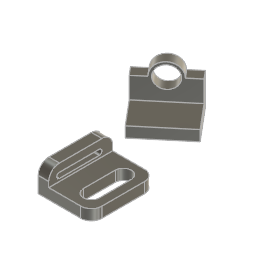
day-5 (Autodesk Fusion 360 design; units mm, degrees)
part number: 2026-04-15-21-22-57-199
Autodesk Fusion 360 part; units mm, degrees
sketch "Sketch1" plane through (0, 0, 0) normal (0, 0, 1) x (1, 0, 0)
  line L0 (0, 0) -> (100, 0)
  line L1 (100, 0) -> (100, -120)
  line L2 (100, -120) -> (0, -120)
  line L3 (0, -120) -> (0, 0)
  dimension "d1" = 100
  dimension "d2" = 120
  constraint horizontal L0
  constraint vertical L1
  constraint horizontal L2
  constraint vertical L3
  constraint coincident L0.start L3.end
  measures "d1" distance of L0.start L0.end
  measures "d2" distance of L0.start L2.end
extrude "Extrude1" add sketch "Sketch1" along normal blind 20 makes body 1
sketch "Sketch2" plane through (0, 0, 0) normal (0, 0, 1) x (1, 0, 0)
  line L0 (83.9736, -28.966) -> (83.9736, -88.966)
  line L1 (53.9736, -88.966) -> (53.9736, -28.966)
  arc A0 (83.9736, -28.966) -> (53.9736, -28.966) centre (68.9736, -28.966) ccw
  arc A1 (53.9736, -88.966) -> (83.9736, -88.966) centre (68.9736, -88.966) ccw
  constraint vertical L0
  constraint vertical L1
extrude "Extrude2" cut sketch "Sketch2" along normal blind 70 bodies 1
sketch "Sketch3" plane through (0, 0, 0) normal (0, 0, 1) x (1, 0, 0)
  line L0 (0, 0) -> (20, 0)
  line L1 (20, 0) -> (20, -120)
  line L2 (20, -120) -> (0, -120)
  line L3 (0, -120) -> (0, 0)
  constraint horizontal L0
  constraint vertical L1
  constraint horizontal L2
  constraint vertical L3
  constraint coincident L0.start L3.end
extrude "Extrude3" add sketch "Sketch3" along normal blind 50 bodies 1
sketch "Sketch4" plane through (0, 0, 0) normal (1, 0, 0) x (0, 1, 0)
  line L0 (-25, 35) -> (-100, 35)
  line L1 (-100, 25) -> (-25, 25)
  arc A0 (-25, 25) -> (-25, 35) centre (-25, 30) ccw
  arc A1 (-100, 35) -> (-100, 25) centre (-100, 30) ccw
  dimension "d14" = 10
  dimension "d15" = 10
  constraint horizontal L0
  constraint horizontal L1
  measures "d14" diameter of A0
  measures "d15" diameter of A1
extrude "Extrude4" cut sketch "Sketch4" along normal blind 25 bodies 1
fillet "Fillet1" radius 20 1 edges at (10, -120, 50) on bodies 1
fillet "Fillet2" radius 20 1 edges at (10, 0, 50) on bodies 1
fillet "Fillet3" radius 20 1 edges at (100, 0, 10) on bodies 1
fillet "Fillet4" radius 20 1 edges at (100, -120, 10) on bodies 1
sketch "Sketch5" plane through (0, 0, 0) normal (0, 0, 1) x (1, 0, 0)
  line L0 (100, 200) -> (100, 140)
  line L1 (100, 140) -> (0, 140)
  line L2 (0, 140) -> (0, 200)
  circle A0 centre (50, 200) radius 20
  arc A1 (75, 200) -> (25, 200) centre (50, 200) ccw
  line L3 (0, 200) -> (25, 200)
  line L4 (75, 200) -> (100, 200)
  dimension "d28" = 40
  dimension "d29" = 50
  constraint horizontal L3
  constraint vertical L0
  constraint horizontal L1
  constraint vertical L2
  constraint concentric A0 A1
  constraint collinear L3 L4
  constraint coincident A0.centre L3
  measures "d28" diameter of A0
  measures "d29" diameter of A1
extrude "Extrude5" add sketch "Sketch5" along normal blind 20 separate body contours L0 L1 L2 A1 L3 L4 | A0 makes body 2
sketch "Sketch6" plane through (0, 0, 20) normal (0, 0, 1) x (-1, 0, 0)
  arc A0 (-75, -200) -> (-25, -200) centre (-50, -200) ccw
  line L0 (-25, -200) -> (0, -200)
  line L1 (0, -200) -> (0, -140)
  line L2 (0, -140) -> (-100, -140)
  line L3 (-100, -140) -> (-100, -200)
  line L4 (-100, -200) -> (-75, -200)
  circle A1 centre (-50, -200) radius 20
  dimension "d32" = 40
  constraint concentric A0 A1
  measures "d32" diameter of A1
extrude "Extrude6" cut sketch "Sketch6" against normal blind 70 contours A1 bodies 2
sketch "Sketch7" plane through (0, 0, 20) normal (0, 0, 1) x (-1, 0, 0)
  circle A0 centre (-50, -200) radius 20
  arc A1 (-75, -200) -> (-25, -200) centre (-50, -200) ccw
  line L0 (-25, -200) -> (0, -200)
  line L1 (0, -200) -> (0, -140)
  line L2 (0, -140) -> (-100, -140)
  line L3 (-100, -140) -> (-100, -200)
  line L4 (-100, -200) -> (-75, -200)
  line L5 (0, -160) -> (-100, -160)
  line L6 (-100, -160) -> (-100, -140)
  line L7 (-100, -140) -> (0, -140)
  line L8 (0, -140) -> (0, -160)
  constraint horizontal L5
  constraint vertical L6
  constraint horizontal L7
  constraint vertical L8
  constraint coincident L1 L5.start
extrude "Extrude7" add sketch "Sketch7" along normal blind 60 contours L1 L2 L3 L5 L6 L7 L8 bodies 2
move_body "Move1" bodies 2 to x (1, 0, 0) y (0, 1, 0) z (0, 0, 1) at (0, -100, 0)
move_body "Move2" bodies 2 to x (0.766044, 0.642788, 0) y (0, 0, 1) z (0.642788, -0.766044, 0) at (-54.4118, 107.8286, -34.2109)
